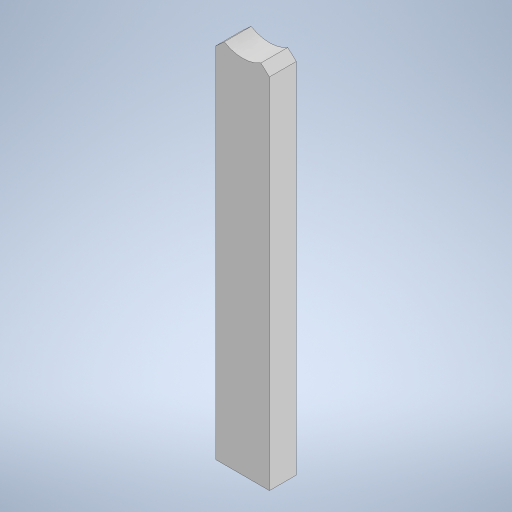
# Autodesk Inventor part: Brazo mdf
Saved by Autodesk Inventor 2023 (Build 270158000, 158)
## iProperties
Created: 2022-10-19
Part Number: Brazo mdf
Material: Generic
Document SubType Name: Modeling
Designer: User
Density: 1 g/cm^3
Appearance: Default
Author: User
Autodesk Inventor part; units mm, degrees
ref_plane "YZ Plane" through (0, 0, 0) normal (1, 0, 0) x (0, 1, 0)
ref_plane "XZ Plane" through (0, 0, 0) normal (0, 1, 0) x (-1, 0, 0)
ref_plane "XY Plane" through (0, 0, 0) normal (0, 0, 1) x (1, 0, 0)
sketch "Sketch2" plane through (0, 0, 0) normal (0, 0, 1) x (1, 0, 0)
  line L0 (-9.9263, 15.061) -> (-14.7098, 10.7077)
  line L1 (-14.7098, 10.7077) -> (-9.9263, 15.061)
  arc A0 (-9.9263, 15.061) -> (10.5068, 15.061) centre (0.2902, 32.2547) ccw
  arc A1 (-9.9263, 15.061) -> (10.5068, 15.061) centre (0.2902, 32.2547) ccw
  line L2 (15.2902, 10.7077) -> (10.5068, 15.061)
  line L3 (15.2902, 10.7077) -> (10.5068, 15.061)
  line L4 (-9.9263, 15.061) -> (10.5068, 15.061) construction
  line L5 (15.2902, 10.7077) -> (15.2902, -189.2923)
  line L6 (-14.7098, 10.7077) -> (-14.7098, -189.2923)
  line L7 (15.2902, -189.2923) -> (-14.7098, -189.2923)
  point P0 (0.741, 0.8123)
  point P1 (0.741, 0.8123)
  dimension "d3" = 137.695
  dimension "d4" = 95.39
  dimension "d5" = 4.3533
  dimension "d15" = 200
  dimension "d16" = 200
  constraints: 16 end point, 4 point on circle, 2 centre point, 2 collinear, 2 horizontal, 2 vertical, 1 coincident
  measures "d3" angle of L2 L4
  measures "d4" angle of L2 L0
  measures "d5" distance from line of L2.start L4
  measures "d15" distance of L2.start L5.end
  measures "d16" distance of L0.end L6.end
extrude "Extrusion1" add sketch "Sketch2" along normal blind 15
body "Solid1"
